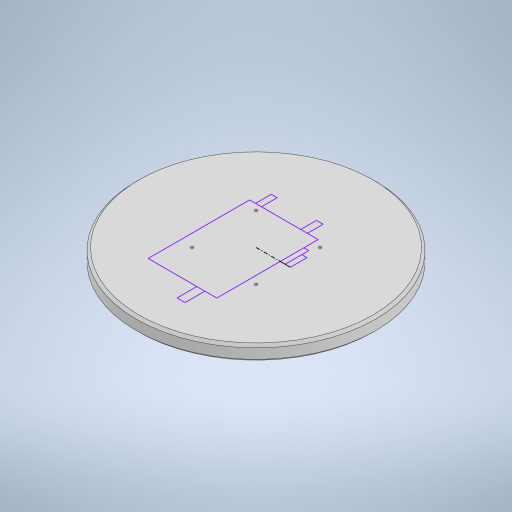
# Autodesk Inventor part: Base_Cap
Saved by Autodesk Inventor 2023 (Build 270158000, 158)
## iProperties
Created: 2025-02-06
Part Number: Base_Cap
Material: Generic
Document SubType Name: Modeling
Designer: Swoby
Density: 1 g/cm^3
Appearance: Default
Author: Swoby
Autodesk Inventor part; units mm, degrees
ref_plane "YZ Plane" through (0, 0, 0) normal (1, 0, 0) x (0, 1, 0)
ref_plane "XZ Plane" through (0, 0, 0) normal (0, 1, 0) x (-1, 0, 0)
ref_plane "XY Plane" through (0, 0, 0) normal (0, 0, 1) x (1, 0, 0)
sketch "Sketch1" plane through (0, 0, 0) normal (0, 0, 1) x (1, 0, 0)
  line L0 (0, 3) -> (0, -3)
  line L1 (0, 3) -> (47.2, 3)
  line L2 (48.2, 2) -> (48.2, -2)
  line L3 (47.2, -3) -> (0, -3)
  line L4 (0, 0) -> (48.2, 0) construction
  line L5 (47.2, 3) -> (48.2, 2)
  line L6 (48.2, -2) -> (47.2, -3)
  point P0 (48.2, 3)
  point P1 (48.2, -3)
  dimension "d0" = 96.4
  dimension "d1" = 6
  dimension "d2" = 1
  dimension "d3" = 1
  dimension "d4" = 1
  dimension "d5" = 1
  constraints: 14 end point, 4 point on line, 3 perpendicular, 2 midpoint, 1 horizontal, 1 vertical
  measures "d0" diameter of L2 L0
  measures "d1" distance of point (48.2, 3) point (48.2, -3)
  measures "d2" distance of L1.end point (48.2, 3)
  measures "d3" distance of L2.start point (48.2, 3)
  measures "d4" distance of L2.end point (48.2, -3)
  measures "d5" distance of L3.start point (48.2, -3)
revolve "Revolution1" add sketch "Sketch1" angle 360 about axis through (0, 3, 0) along (0, -1, 0)
sketch "Sketch2" plane through (0, -3, 0) normal (0, -1, 0) x (1, 0, 0)
  circle A0 centre (0, 0) radius 47.2 projected
  line L0 (0, 0) -> (47.2, 0) construction
  line L1 (0, 0) -> (12.9047, -12.9047) construction
  line L2 (0, 0) -> (-12.9047, -12.9047) construction
  arc A1 (11.7375, -14.5288) -> (14.3189, -14.3189) centre (12.9047, -12.9047) ccw
  arc A2 (-14.3189, -14.3189) -> (-11.7375, -14.5288) centre (-12.9047, -12.9047) ccw
  line L3 (4.5962, -4.5962) -> (1.8031, -7.3893) construction
  line L4 (-4.5962, -4.5962) -> (-1.8031, -7.3893) construction
  line L5 (12.9047, -12.9047) -> (14.3189, -14.3189) construction
  line L6 (-12.9047, -12.9047) -> (-14.3189, -14.3189) construction
  line L7 (-1.8031, -7.3893) -> (-11.7375, -14.5288)
  line L8 (1.8031, -7.3893) -> (11.7375, -14.5288)
  arc A3 (1.8031, -7.3893) -> (-1.8031, -7.3893) centre (0, -9.8982) ccw
  line L9 (4.5962, 4.5962) -> (7.3893, 1.8031) construction
  line L10 (7.3893, 1.8031) -> (14.5288, 11.7375)
  line L11 (12.9047, 12.9047) -> (14.3189, 14.3189) construction
  arc A4 (14.5288, 11.7375) -> (14.3189, 14.3189) centre (12.9047, 12.9047) ccw
  arc A5 (7.3893, 1.8031) -> (7.3893, -1.8031) centre (9.8982, 0) ccw
  line L12 (4.5962, -4.5962) -> (7.3893, -1.8031) construction
  line L13 (7.3893, -1.8031) -> (14.5288, -11.7375)
  arc A6 (14.3189, -14.3189) -> (14.5288, -11.7375) centre (12.9047, -12.9047) ccw
  line L14 (12.9047, -12.9047) -> (14.3189, -14.3189) construction
  line L15 (-4.5962, 4.5962) -> (-1.8031, 7.3893) construction
  line L16 (-1.8031, 7.3893) -> (-11.7375, 14.5288)
  line L17 (-12.9047, 12.9047) -> (-14.3189, 14.3189) construction
  arc A7 (-11.7375, 14.5288) -> (-14.3189, 14.3189) centre (-12.9047, 12.9047) ccw
  arc A8 (-1.8031, 7.3893) -> (1.8031, 7.3893) centre (0, 9.8982) ccw
  line L18 (4.5962, 4.5962) -> (1.8031, 7.3893) construction
  line L19 (1.8031, 7.3893) -> (11.7375, 14.5288)
  arc A9 (14.3189, 14.3189) -> (11.7375, 14.5288) centre (12.9047, 12.9047) ccw
  line L20 (12.9047, 12.9047) -> (14.3189, 14.3189) construction
  line L21 (-4.5962, -4.5962) -> (-7.3893, -1.8031) construction
  line L22 (-7.3893, -1.8031) -> (-14.5288, -11.7375)
  line L23 (-12.9047, -12.9047) -> (-14.3189, -14.3189) construction
  arc A10 (-14.5288, -11.7375) -> (-14.3189, -14.3189) centre (-12.9047, -12.9047) ccw
  arc A11 (-7.3893, -1.8031) -> (-7.3893, 1.8031) centre (-9.8982, 0) ccw
  line L24 (-4.5962, 4.5962) -> (-7.3893, 1.8031) construction
  line L25 (-7.3893, 1.8031) -> (-14.5288, 11.7375)
  arc A12 (-14.3189, 14.3189) -> (-14.5288, 11.7375) centre (-12.9047, 12.9047) ccw
  line L26 (-12.9047, 12.9047) -> (-14.3189, 14.3189) construction
  point P0 (0, 0)
  dimension "d7" = 45
  dimension "d8" = 18.25
  dimension "d9" = 18.25
  dimension "d10" = 4
  dimension "d11" = 4
  dimension "d13" = 6.5
  dimension "d14" = 6.5
  dimension "d15" = 3.95
  dimension "d16" = 3.95
  dimension "d19" = 360
  constraints: 54 end point, 24 point on circle, 12 centre point, 8 coincident, 3 perpendicular, 3 tangent, 2 collinear, 2 point on line, 1 horizontal, 1 horizontal alignment, 90 other
  measures "d7" angle of L0 L1
  measures "d8" distance of L0.start L1.end
  measures "d9" distance of L0.start L2.end
  measures "d10" diameter of A1
  measures "d11" diameter of A2
  measures "d13" distance from line of point (0, 0) L3
  measures "d14" distance from line of point (0, 0) L4
  measures "d15" distance of L4.start L4.end
  measures "d16" distance of L3.start L3.end
extrude "Extrusion1" cut sketch "Sketch2" against normal blind 4 contours L8 A3 L7 A2 A10 L22 A11 L25 A12 A7 L16 A8 L19 A9 A4 L10 A5 L13 A6 A1
sketch "Sketch3" plane through (0, 1, 0) normal (0, -1, 0) x (1, 0, 0)
  arc A0 (11.7375, -14.5288) -> (14.5288, -11.7375) centre (12.9047, -12.9047) ccw projected
  line L0 (7.3893, -1.8031) -> (14.5288, -11.7375) projected
  arc A1 (7.3893, 1.8031) -> (7.3893, -1.8031) centre (9.8982, 0) ccw projected
  line L1 (14.5288, 11.7375) -> (7.3893, 1.8031) projected
  arc A2 (14.5288, 11.7375) -> (11.7375, 14.5288) centre (12.9047, 12.9047) ccw projected
  line L2 (1.8031, 7.3893) -> (11.7375, 14.5288) projected
  arc A3 (-1.8031, 7.3893) -> (1.8031, 7.3893) centre (0, 9.8982) ccw projected
  line L3 (-11.7375, 14.5288) -> (-1.8031, 7.3893) projected
  arc A4 (-11.7375, 14.5288) -> (-14.5288, 11.7375) centre (-12.9047, 12.9047) ccw projected
  line L4 (-7.3893, 1.8031) -> (-14.5288, 11.7375) projected
  arc A5 (-7.3893, -1.8031) -> (-7.3893, 1.8031) centre (-9.8982, 0) ccw projected
  line L5 (-14.5288, -11.7375) -> (-7.3893, -1.8031) projected
  arc A6 (-14.5288, -11.7375) -> (-11.7375, -14.5288) centre (-12.9047, -12.9047) ccw projected
  line L6 (-1.8031, -7.3893) -> (-11.7375, -14.5288) projected
  arc A7 (1.8031, -7.3893) -> (-1.8031, -7.3893) centre (0, -9.8982) ccw projected
  line L7 (11.7375, -14.5288) -> (1.8031, -7.3893) projected
  circle A8 centre (-12.9047, 12.9047) radius 0.5
  circle A9 centre (-12.9047, -12.9047) radius 0.5
  circle A10 centre (12.9047, -12.9047) radius 0.5
  circle A11 centre (12.9047, 12.9047) radius 0.5
  point P0 (0, 0)
  dimension "d23" = 1
  dimension "d24" = 1
  dimension "d25" = 1
  dimension "d26" = 1
  constraints: 4 centre point, 4 coincident
  measures "d23" diameter of A8
  measures "d24" diameter of A9
  measures "d25" diameter of A10
  measures "d26" diameter of A11
extrude "Extrusion2" cut sketch "Sketch3" against normal blind 6 contours A8 | A9 | A10 | A11
sketch "Sketch4" plane through (0, 3, 0) normal (0, 1, 0) x (1, 0, 0)
  line L0 (0, 0) -> (11.2714, 0)
  line L1 (9.7111, 15.2948) -> (-17.9468, 15.2948)
  line L2 (-17.9468, 15.2948) -> (-17.9468, -25.581)
  line L3 (-17.9468, -25.581) -> (9.7111, -25.581)
  line L4 (9.7111, -25.581) -> (9.7111, 15.2948)
  line L5 (11.6724, 9.5312) -> (9.7111, 9.5312)
  line L6 (9.7111, 9.5312) -> (9.7111, 0)
  line L7 (9.7111, 0) -> (11.6724, 0)
  line L8 (11.6724, 0) -> (11.6724, 9.5312)
  line L9 (13.7771, 6.7249) -> (11.6724, 6.7249)
  line L10 (11.6724, 6.7249) -> (11.6724, 0)
  line L11 (11.6724, 0) -> (13.7771, 0)
  line L12 (13.7771, 0) -> (13.7771, 6.7249)
  line L13 (2.6923, 15.2948) -> (5.3583, 15.2948)
  line L14 (5.3583, 15.2948) -> (5.3583, 21.6449)
  line L15 (5.3583, 21.6449) -> (2.6923, 21.6449)
  line L16 (2.6923, 21.6449) -> (2.6923, 15.2948)
  line L17 (1.6633, -25.581) -> (4.8906, -25.581)
  line L18 (4.8906, -25.581) -> (4.8906, -33.5452)
  line L19 (4.8906, -33.5452) -> (1.6633, -33.5452)
  line L20 (1.6633, -33.5452) -> (1.6633, -25.581)
  line L21 (-15.5485, 15.2948) -> (-13.1631, 15.2948)
  line L22 (-13.1631, 15.2948) -> (-13.1631, 21.6449)
  line L23 (-13.1631, 21.6449) -> (-15.5485, 21.6449)
  line L24 (-15.5485, 21.6449) -> (-15.5485, 15.2948)
  constraints: 50 end point, 12 parallel, 7 horizontal, 6 perpendicular, 6 point on line
equation "\"d3\" = d2"
equation "\"d4\" = d2"
equation "\"d5\" = d4"
equation "\"d9\" = d8"
body "Solid1"
